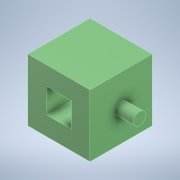
# Autodesk Inventor part: prismaticFulcrum
Saved by Autodesk Inventor 2022 (Build 260153000, 153)
## iProperties
Created: 2021-12-27
Part Number: prismaticFulcrum
Material: Generic
Document SubType Name: Modeling
Designer: G S SHOURIE
Density: 1 g/cm^3
Appearance: Smooth - Dark Forest Green
Author: G S SHOURIE
Autodesk Inventor part; units mm, degrees
ref_plane "YZ Plane" through (0, 0, 0) normal (1, 0, 0) x (0, 1, 0)
ref_plane "XZ Plane" through (0, 0, 0) normal (0, 1, 0) x (-1, 0, 0)
ref_plane "XY Plane" through (0, 0, 0) normal (0, 0, 1) x (1, 0, 0)
sketch "Sketch1" plane through (0, 0, 0) normal (0, 0, 1) x (1, 0, 0)
  line L0 (-25, 25) -> (25, 25)
  line L1 (25, 25) -> (25, -25)
  line L2 (25, -25) -> (-25, -25)
  line L3 (-25, -25) -> (-25, 25)
  line L4 (-10, 10) -> (10, 10)
  line L5 (10, 10) -> (10, -10)
  line L6 (10, -10) -> (-10, -10)
  line L7 (-10, -10) -> (-10, 10)
  point P0 (0, 0)
  dimension "d0" = 50
  dimension "d1" = 50
  dimension "d2" = 25
  dimension "d3" = 25
  dimension "d4" = 20
  dimension "d5" = 20
  dimension "d6" = 10
  dimension "d7" = 10
  constraints: 16 end point, 4 parallel, 2 horizontal, 2 perpendicular
  measures "d0" distance of L0.end L1.end
  measures "d1" distance of L0.start L0.end
  measures "d2" distance from line of L3 point (0, 0)
  measures "d3" distance from line of L0 point (0, 0)
  measures "d4" distance of L4.end L5.end
  measures "d5" distance of L4.start L4.end
  measures "d6" distance from line of L4 point (0, 0)
  measures "d7" distance from line of L7 point (0, 0)
extrude "Extrusion1" add sketch "Sketch1" along normal mid plane 50
sketch "Sketch2" plane through (-25, -25, 25) normal (-1, 0, 0) x (0, 0, 1)
  circle A0 centre (-25, 25) radius 5
  dimension "d10" = 10
  constraints: 1 centre point, 1 coincident
  measures "d10" diameter of A0
extrude "Extrusion2" add sketch "Sketch2" along normal blind 15
mirror "Mirror1" about plane through (0, 0, 0) normal (1, 0, 0) of "Extrusion2"
body "Solid1"
